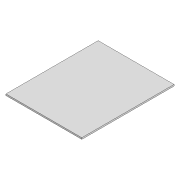
# Autodesk Inventor part: base
Saved by Autodesk Inventor 2020 (Build 240168000, 168)
## iProperties
Created: 2021-09-21
Part Number: base
Material: Generic
Document SubType Name: Modeling
Designer: pablo
Density: 1 g/cm^3
Appearance: Default
Author: pablo
Autodesk Inventor part; units mm, degrees
ref_plane "YZ Plane" through (0, 0, 0) normal (1, 0, 0) x (0, 1, 0)
ref_plane "XZ Plane" through (0, 0, 0) normal (0, 1, 0) x (-1, 0, 0)
ref_plane "XY Plane" through (0, 0, 0) normal (0, 0, 1) x (1, 0, 0)
sketch "Sketch1" plane through (0, 0, 0) normal (0, 1, 0) x (-1, 0, 0)
  line L0 (127.5, -155) -> (-127.5, -155)
  line L1 (-127.5, -155) -> (-127.5, 155)
  line L2 (-127.5, 155) -> (127.5, 155)
  line L3 (127.5, 155) -> (127.5, -155)
  line L4 (127.5, -155) -> (-127.5, 155) construction
  line L5 (-127.5, -155) -> (127.5, 155) construction
  point P0 (0, 0)
  dimension "d0" = 255
  dimension "d1" = 310
  constraints: 12 end point, 2 midpoint, 2 parallel, 1 horizontal, 1 perpendicular
  measures "d0" distance of L1.end L2.end
  measures "d1" distance of L0.end L1.end
extrude "Extrusion1" add sketch "Sketch1" along normal blind 5
body "Solid1"
